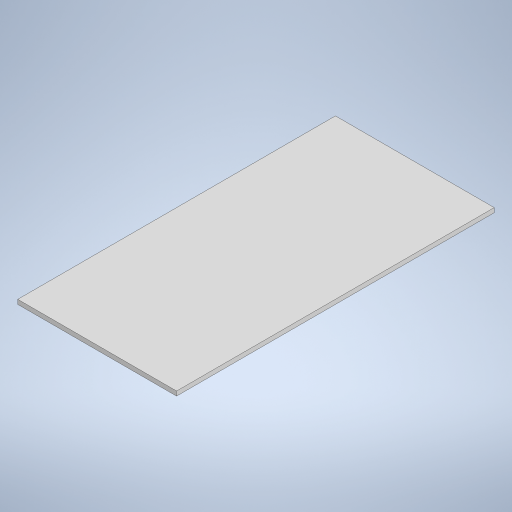
# Autodesk Inventor part: 6'x3' plywood
Saved by Autodesk Inventor 2023 (Build 270158000, 158)
## iProperties
Created: 2022-08-18
Part Number: 6'x3' plywood
Material: Generic
Document SubType Name: Modeling
Designer: rkant
Density: 1 g/cm^3
Appearance: Default
Author: rkant
Autodesk Inventor part; units mm, degrees
ref_plane "YZ Plane" through (0, 0, 0) normal (1, 0, 0) x (0, 1, 0)
ref_plane "XZ Plane" through (0, 0, 0) normal (0, 1, 0) x (-1, 0, 0)
ref_plane "XY Plane" through (0, 0, 0) normal (0, 0, 1) x (1, 0, 0)
sketch "Sketch1" plane through (0, 0, 0) normal (0, 1, 0) x (-1, 0, 0)
  line L0 (-457.2, 914.4) -> (457.2, 914.4)
  line L1 (457.2, 914.4) -> (457.2, -914.4)
  line L2 (457.2, -914.4) -> (-457.2, -914.4)
  line L3 (-457.2, -914.4) -> (-457.2, 914.4)
  line L4 (-457.2, 914.4) -> (457.2, -914.4) construction
  line L5 (457.2, 914.4) -> (-457.2, -914.4) construction
  point P0 (0, 0)
  dimension "d0" = 914.4
  dimension "d1" = 1828.8
  constraints: 12 end point, 2 midpoint, 2 parallel, 1 horizontal, 1 perpendicular
  measures "d0" distance of L0.start L0.end
  measures "d1" distance of L0.end L1.end
extrude "Extrusion1" add sketch "Sketch1" along normal blind 25.4
body "Solid1"
